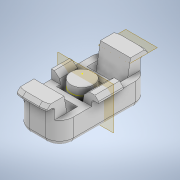
# Autodesk Inventor part: ps3buttonr1
Saved by Autodesk Inventor 2021 (Build 250183000, 183)
## iProperties
Created: 2023-05-05
Part Number: ps3buttonr1
Material: Generic
Document SubType Name: Modeling
Designer: assman
Density: 1 g/cm^3
Appearance: Default
Author: assman
## iProperties of the stored document _3DPrint.ipt
Created: 2023-05-05
Part Number: _3DPrint
Material: Generic
Document SubType Name: Modeling
Designer: assman
Density: 1 g/cm^3
Appearance: Default
Author: assman
Autodesk Inventor part; units mm, degrees
ref_plane "YZ Plane" through (0, 0, 0) normal (1, 0, 0) x (0, 1, 0)
ref_plane "XZ Plane" through (0, 0, 0) normal (0, 1, 0) x (-1, 0, 0)
sketch "Sketch1" plane through (0, 0, 0) normal (0, 1, 0) x (-1, 0, 0)
  line L0 (1.825, 9.85) -> (-1.825, 9.85)
  line L1 (-4.825, 6.85) -> (-4.825, -6.85)
  line L2 (-1.825, -9.85) -> (1.825, -9.85)
  line L3 (4.825, -6.85) -> (4.825, 6.85)
  line L4 (4.825, 9.85) -> (-4.825, -9.85) construction
  line L5 (-4.825, 9.85) -> (4.825, -9.85) construction
  arc A0 (4.825, 6.85) -> (1.825, 9.85) centre (1.825, 6.85) ccw
  arc A1 (1.825, -9.85) -> (4.825, -6.85) centre (1.825, -6.85) ccw
  arc A2 (-4.825, -6.85) -> (-1.825, -9.85) centre (-1.825, -6.85) ccw
  arc A3 (-1.825, 9.85) -> (-4.825, 6.85) centre (-1.825, 6.85) ccw
  point P0 (0, 0)
  dimension "d0" = 9.65
  dimension "d1" = 19.7
  dimension "d2" = 3
  constraints: 12 end point, 8 point on circle, 8 point on line, 8 tangent, 4 centre point, 3 equal radius, 2 midpoint, 2 parallel, 1 horizontal, 1 perpendicular
  measures "d0" distance of L5.end L4.end
  measures "d1" distance of L4.end L5.start
  measures "d2" radius of A0
extrude "Extrusion1" add sketch "Sketch1" along normal blind 5
sketch "Sketch2" plane through (0, 5, 0) normal (0, 1, 0) x (1, 0, 0)
  arc A0 (1.825, -9.85) -> (4.825, -6.85) centre (1.825, -6.85) ccw projected
  line L0 (4.825, -6.85) -> (4.825, 6.85) projected
  arc A1 (4.825, 6.85) -> (1.825, 9.85) centre (1.825, 6.85) ccw projected
  line L1 (1.825, 9.85) -> (-1.825, 9.85) projected
  arc A2 (-1.825, 9.85) -> (-4.825, 6.85) centre (-1.825, 6.85) ccw projected
  line L2 (-4.825, 6.85) -> (-4.825, -6.85) projected
  arc A3 (-4.825, -6.85) -> (-1.825, -9.85) centre (-1.825, -6.85) ccw projected
  line L3 (-1.825, -9.85) -> (1.825, -9.85) projected
  line L4 (-3.825, -8.85) -> (-3.825, 8.85)
  line L5 (-3.825, 8.85) -> (3.825, 8.85)
  line L6 (3.825, 8.85) -> (3.825, -8.85)
  line L7 (3.825, -8.85) -> (-3.825, -8.85)
  line L8 (0, -8.85) -> (0, -3.85) construction
  line L9 (0, -3.85) -> (0, -2.85) construction
  line L10 (-3.825, -2.85) -> (3.825, -2.85)
  line L11 (3.825, -2.85) -> (3.825, 2.85)
  line L12 (3.825, 2.85) -> (-3.825, 2.85)
  line L13 (-3.825, 2.85) -> (-3.825, -2.85)
  line L14 (-3.825, -2.85) -> (3.825, 2.85) construction
  line L15 (3.825, -2.85) -> (-3.825, 2.85) construction
  line L16 (-3.825, 3.85) -> (3.825, 3.85)
  line L17 (3.825, 3.85) -> (3.825, 8.85)
  line L18 (3.825, 8.85) -> (-3.825, 8.85)
  line L19 (-3.825, 8.85) -> (-3.825, 3.85)
  line L20 (-3.825, 3.85) -> (3.825, 8.85) construction
  line L21 (3.825, 3.85) -> (-3.825, 8.85) construction
  line L22 (-3.825, -8.85) -> (3.825, -8.85)
  line L23 (3.825, -8.85) -> (3.825, -3.85)
  line L24 (3.825, -3.85) -> (-3.825, -3.85)
  line L25 (-3.825, -3.85) -> (-3.825, -8.85)
  line L26 (-3.825, -8.85) -> (3.825, -3.85) construction
  line L27 (3.825, -8.85) -> (-3.825, -3.85) construction
  point P0 (0, 0)
  point P1 (0, 6.35)
  point P2 (0, -6.35)
  dimension "d5" = 1
  dimension "d6" = 5
  dimension "d8" = 1
  constraints: 48 end point, 8 midpoint, 6 parallel, 3 horizontal, 3 perpendicular, 2 point on line, 2 vertical, 3 other
  measures "d5" distance between parallel lines of L2 L4
  measures "d6" distance of L8.start L8.end
  measures "d8" distance of L8.end L9.end
extrude "Extrusion2" cut sketch "Sketch2" against normal blind 3.94 contours L4 L24 L6 L7 | L4 L12 L6 L10 | L4 L5 L6 L16
sketch "Sketch4" plane through (0, 1.06, 0) normal (0, 1, 0) x (1, 0, 0)
  line L0 (-3.825, -2.85) -> (-3.825, 2.85) construction
  line L1 (3.825, -2.85) -> (-3.825, -2.85) construction
  line L2 (3.825, 2.85) -> (3.825, -2.85) construction
  line L3 (-3.825, 2.85) -> (3.825, 2.85) construction
  circle A0 centre (0, 0) radius 2.5
  dimension "d14" = 5
  constraints: 1 centre point, 1 coincident
  measures "d14" diameter of A0
extrude "Extrusion3" add sketch "Sketch4" along normal up to surface (3.94 mm away)
sketch "Sketch5" plane through (0, 5, 0) normal (0, 1, 0) x (1, 0, 0)
  circle A0 centre (0, 0) radius 2.5 projected
thicken "Thicken1" operation add thickness 1.6 both sides no extend neighbours yes toward (0, 1, 0) faces at (1.2612, 5, 0.6619)
fillet "Fillet1" radius 1 1 edges at (-2.5, 1.06, 0)
thicken "Thicken2" operation add thickness 0.5 both sides no extend neighbours yes toward (0, 0, -1) faces at (-1.275, 3.6867, 8.85) (-3.825, 3.6867, 5.5167) (1.275, 3.6867, 3.85) (3.825, 2.3733, 5.5167)
thicken "Thicken3" operation add thickness 0.5 both sides no extend neighbours yes toward (1, 0, 0) faces at (-3.825, 2.3733, -5.5167) (1.275, 3.6867, -8.85) (3.825, 2.3733, -7.1833) (-1.275, 3.6867, -3.85)
sketch "Sketch6" plane through (1.825, 0, -9.85) normal (0, 0, -1) x (-1, 0, 0)
  line L0 (0, 0) -> (3.65, 0) construction
  line L1 (3.65, 0) -> (3.65, 5) construction
  line L2 (0, 5) -> (3.65, 5) construction
  line L3 (0, 0) -> (0, 5) construction
  line L4 (3.65, 5) -> (0, 5) construction
  line L5 (1.825, 5) -> (1.825, 0) construction
  line L6 (-0.175, 6.75) -> (3.825, 6.75) construction
  line L7 (3.825, 6.75) -> (3.825, 3.25) construction
  line L8 (3.825, 3.25) -> (-0.175, 3.25) construction
  line L9 (-0.175, 3.25) -> (-0.175, 6.75) construction
  line L10 (-0.175, 6.75) -> (3.825, 3.25) construction
  line L11 (3.825, 6.75) -> (-0.175, 3.25) construction
  line L12 (-0.175, 5) -> (5.825, 5)
  line L13 (5.825, 5) -> (5.825, 8.5)
  line L14 (5.825, 8.5) -> (-0.175, 8.5)
  line L15 (-0.175, 8.5) -> (-0.175, 5)
  dimension "d21" = 4
  dimension "d22" = 3.5
  dimension "d26" = 3.5
  constraints: 22 end point, 4 midpoint, 4 parallel, 2 horizontal, 2 perpendicular, 1 vertical
  measures "d21" distance of L7.end L8.end
  measures "d22" distance of L6.end L7.end
  measures "d26" distance of L13.end L12.end
extrude "Extrusion5" [suppressed]
sketch "Sketch8" plane through (1.825, 0, -9.85) normal (0, 0, -1) x (-1, 0, 0)
  line L0 (0, 0) -> (3.65, 0) construction
  line L1 (3.65, 0) -> (3.65, 5) construction
  line L2 (0, 0) -> (0, 5) construction
  line L3 (-0.175, 8.5) -> (-0.175, 5) projected
  line L4 (5.825, 8.5) -> (5.825, 5) projected
  line L5 (-0.175, 8.5) -> (5.825, 8.5)
  line L6 (5.825, 8.5) -> (5.825, 7.11)
  line L7 (5.825, 7.11) -> (-0.175, 7.11)
  line L8 (-0.175, 7.11) -> (-0.175, 8.5)
  line L9 (0, 5) -> (3.65, 5) projected
  point P0 (1.825, 0)
  point P1 (1.825, 5)
  point P2 (-0.175, 7.11)
  dimension "d29" = 1.39
  constraints: 8 end point, 2 parallel, 1 horizontal, 1 perpendicular, 1 point on line, 1 other
  measures "d29" distance of L5.end L6.end
extrude "Extrusion6" [suppressed]
chamfer "Chamfer1" [suppressed]
sketch "Sketch9" plane through (1.825, 0, -9.85) normal (0, 0, -1) x (-1, 0, 0)
  line L0 (0, 0) -> (0, 5) construction
  line L1 (0, 0) -> (3.65, 0) construction
  line L2 (3.65, 0) -> (3.65, 5) construction
  line L3 (1.825, 5) -> (0.825, 5)
  line L4 (0.825, 5) -> (0.825, 3)
  line L5 (0.825, 3) -> (1.825, 3)
  line L6 (1.825, 3) -> (1.825, 5)
  line L7 (5.825, 5) -> (6.825, 5)
  line L8 (6.825, 5) -> (6.825, 3)
  line L9 (6.825, 3) -> (5.825, 3)
  line L10 (5.825, 3) -> (5.825, 5)
  line L11 (0, 5) -> (3.65, 5) projected
  point P0 (1.825, 0)
  dimension "d35" = 1
  dimension "d36" = 2
  dimension "d37" = 1
  dimension "d38" = 2
  constraints: 16 end point, 4 parallel, 2 horizontal, 2 perpendicular
  measures "d35" distance of L5.end L4.end
  measures "d36" distance of L4.end L3.end
  measures "d37" distance of L8.end L9.end
  measures "d38" distance of L7.end L8.end
extrude "Extrusion7" [suppressed]
mirror "Mirror1" [suppressed]
sketch "Sketch10" plane through (4.825, 0, 6.85) normal (1, 0, 0) x (0, 0, -1)
  line L0 (0, 0) -> (13.7, 0) construction
  line L1 (13.7, 0) -> (13.7, 5) construction
  line L2 (0, 5) -> (13.7, 5) construction
  line L3 (0, 0) -> (0, 5) construction
  line L4 (8.85, 4.7327) -> (8.85, 0.7758) construction
  line L5 (6.625, 4.6249) -> (11.075, 4.6249) construction
  line L6 (11.075, 4.6249) -> (11.075, 2.1249) construction
  line L7 (11.075, 2.1249) -> (6.625, 2.1249) construction
  line L8 (6.625, 2.1249) -> (6.625, 4.6249) construction
  line L9 (6.625, 4.6249) -> (11.075, 2.1249) construction
  line L10 (11.075, 4.6249) -> (6.625, 2.1249) construction
  line L11 (6.625, 5) -> (11.075, 5)
  line L12 (11.075, 5) -> (11.075, 7.5)
  line L13 (11.075, 7.5) -> (6.625, 7.5)
  line L14 (6.625, 7.5) -> (6.625, 5)
  point P0 (6.85, 0)
  point P1 (8.85, 3.3749)
  dimension "d41" = 4.45
  dimension "d42" = 2.5
  dimension "d43" = 4.45
  dimension "d44" = 2.5
  constraints: 22 end point, 4 parallel, 3 point on line, 2 horizontal, 2 midpoint, 2 perpendicular, 1 vertical
  measures "d41" distance of L6.end L7.end
  measures "d42" distance of L5.end L6.end
  measures "d43" distance of L13.end L12.end
  measures "d44" distance of L12.end L11.end
extrude "Extrusion8" [suppressed]
sketch "Sketch11" plane through (4.825, 0, 6.85) normal (1, 0, 0) x (0, 0, -1)
  line L0 (0, 0) -> (13.7, 0) construction
  line L1 (13.7, 0) -> (13.7, 5) construction
  line L2 (0, 5) -> (13.7, 5) construction
  line L3 (0, 0) -> (0, 5) construction
  line L4 (6.625, 5) -> (5.825, 5)
  line L5 (5.825, 5) -> (5.825, 3)
  line L6 (5.825, 3) -> (6.625, 3)
  line L7 (6.625, 3) -> (6.625, 5)
  line L8 (11.075, 5) -> (11.875, 5)
  line L9 (11.875, 5) -> (11.875, 3)
  line L10 (11.875, 3) -> (11.075, 3)
  line L11 (11.075, 3) -> (11.075, 5)
  point P0 (6.85, 0)
  dimension "d47" = 0.8
  dimension "d48" = 2
  dimension "d49" = 0.8
  dimension "d50" = 2
  constraints: 16 end point, 4 parallel, 2 horizontal, 2 perpendicular
  measures "d47" distance of L6.end L5.end
  measures "d48" distance of L5.end L4.end
  measures "d49" distance of L9.end L10.end
  measures "d50" distance of L8.end L9.end
extrude "Extrusion9" [suppressed]
sketch "Sketch12" plane through (4.825, 0, 6.85) normal (1, 0, 0) x (0, 0, -1)
  line L0 (0, 5) -> (13.7, 5) construction
  line L1 (0, 0) -> (0, 5) construction
  line L2 (0, 0) -> (13.7, 0) construction
  line L3 (13.7, 0) -> (13.7, 5) construction
  line L4 (6.625, 7.5) -> (11.075, 7.5) projected
  line L5 (11.075, 3) -> (11.075, 7.5) projected
  line L6 (6.625, 7.5) -> (11.075, 7.5)
  line L7 (11.075, 7.5) -> (11.075, 6)
  line L8 (11.075, 6) -> (6.625, 6)
  line L9 (6.625, 6) -> (6.625, 7.5)
  point P0 (6.85, 0)
  dimension "d53" = 1.5
  constraints: 8 end point, 2 parallel, 1 horizontal, 1 perpendicular, 1 point on line
  measures "d53" distance of L6.end L7.end
extrude "Extrusion10" [suppressed]
chamfer "Chamfer2" [suppressed]
sketch "Sketch13" plane through (-4.825, 0, -6.85) normal (-1, 0, 0) x (0, 0, 1)
  line L0 (0, 0) -> (13.7, 0) construction
  line L1 (13.7, 0) -> (13.7, 5) construction
  line L2 (0, 5) -> (13.7, 5) construction
  line L3 (0, 0) -> (0, 5) construction
  line L4 (0, 5) -> (13.7, 5) construction
  line L5 (6.85, 5) -> (6.85, 0) construction
  line L6 (5.35, 4.8143) -> (8.35, 4.8143) construction
  line L7 (8.35, 4.8143) -> (8.35, 2.8143) construction
  line L8 (8.35, 2.8143) -> (5.35, 2.8143) construction
  line L9 (5.35, 2.8143) -> (5.35, 4.8143) construction
  line L10 (5.35, 4.8143) -> (8.35, 2.8143) construction
  line L11 (8.35, 4.8143) -> (5.35, 2.8143) construction
  line L12 (5.35, 5) -> (10.35, 5)
  line L13 (10.35, 5) -> (10.35, 7)
  line L14 (10.35, 7) -> (5.35, 7)
  line L15 (5.35, 7) -> (5.35, 5)
  point P0 (6.85, 3.8143)
  dimension "d59" = 3
  dimension "d60" = 2
  dimension "d61" = 2
  constraints: 22 end point, 4 parallel, 3 midpoint, 3 point on line, 2 horizontal, 2 perpendicular, 1 vertical
  measures "d59" distance of L7.end L8.end
  measures "d60" distance of L6.end L7.end
  measures "d61" distance of L13.end L12.end
extrude "Extrusion11" [suppressed]
sketch "Sketch15" plane through (4.825, 0, 6.85) normal (1, 0, 0) x (0, 0, -1)
  line L0 (0, 0) -> (13.7, 0) construction
  line L1 (13.7, 0) -> (13.7, 5) construction
  line L2 (0, 5) -> (13.7, 5) construction
  line L3 (0, 0) -> (0, 5) construction
  line L4 (4.35, 6.6) -> (9.35, 6.6) construction
  line L5 (4.35, 2.06) -> (9.35, 2.06) construction
  line L6 (4, 5) -> (4, 1.06) construction
  line L7 (9.7, 5) -> (4, 5) construction
  line L8 (9.7, 5) -> (9.7, 1.06) construction
  line L9 (4.625, 6) -> (9.075, 6) construction
  line L10 (9.075, 6) -> (9.075, 4) construction
  line L11 (9.075, 4) -> (4.625, 4) construction
  line L12 (4.625, 4) -> (4.625, 6) construction
  line L13 (9.7, 5) -> (4, 5) construction
  line L14 (4.625, 6) -> (9.075, 4) construction
  line L15 (9.075, 6) -> (4.625, 4) construction
  line L16 (4.625, 5) -> (9.075, 5)
  line L17 (9.075, 5) -> (9.075, 7.5)
  line L18 (9.075, 7.5) -> (4.625, 7.5)
  line L19 (4.625, 7.5) -> (4.625, 5)
  line L20 (9.7, 1.06) -> (4, 1.06) projected
  point P0 (6.85, 0)
  point P1 (6.85, 5)
  dimension "d70" = 4.45
  dimension "d71" = 2
  dimension "d72" = 2.5
  dimension "d97" = 4.45
  constraints: 20 end point, 4 midpoint, 4 parallel, 2 horizontal, 2 perpendicular, 1 point on line
  measures "d70" distance of L10.end L11.end
  measures "d71" distance of L9.end L10.end
  measures "d72" distance of L17.end L16.end
  measures "d97" distance of L17.end L18.end
extrude "Extrusion13" add sketch "Sketch15" against normal up to surface (1 mm away)
thicken "Thicken4" operation add thickness 0.5 both sides no extend neighbours yes toward (-1, 0, 0) faces at (3.825, 2.3733, -0.7417)
draft "FaceDraft1" angle 10 pull direction (0, 1, 0) faces at (3.325, 3.6918, 0) fixed edges at (3.325, 7.5, 0)
sketch "Sketch16" plane through (-4.825, 0, -6.85) normal (-1, 0, 0) x (0, 0, 1)
  line L0 (0, 0) -> (13.7, 0) construction
  line L1 (13.7, 0) -> (13.7, 5) construction
  line L2 (0, 5) -> (13.7, 5) construction
  line L3 (0, 0) -> (0, 5) construction
  line L4 (9.7, 5) -> (4, 5) construction
  line L5 (9.7, 5) -> (9.7, 1.06) construction
  line L6 (9.7, 1.06) -> (4, 1.06) construction
  line L7 (4, 5) -> (4, 1.06) construction
  line L8 (5.35, 6) -> (8.35, 6) construction
  line L9 (8.35, 6) -> (8.35, 4) construction
  line L10 (8.35, 4) -> (5.35, 4) construction
  line L11 (5.35, 4) -> (5.35, 6) construction
  line L12 (9.7, 5) -> (4, 5) construction
  line L13 (5.35, 6) -> (8.35, 4) construction
  line L14 (8.35, 6) -> (5.35, 4) construction
  line L15 (5.35, 5) -> (8.35, 5)
  line L16 (8.35, 5) -> (8.35, 7)
  line L17 (8.35, 7) -> (5.35, 7)
  line L18 (5.35, 7) -> (5.35, 5)
  point P0 (6.85, 0)
  point P1 (6.85, 5)
  dimension "d78" = 3
  dimension "d79" = 2
  dimension "d80" = 2
  constraints: 20 end point, 4 midpoint, 4 parallel, 2 horizontal, 2 perpendicular, 1 point on line
  measures "d78" distance of L9.end L10.end
  measures "d79" distance of L8.end L9.end
  measures "d80" distance of L16.end L15.end
extrude "Extrusion14" add sketch "Sketch16" against normal up to surface (1 mm away)
thicken "Thicken5" operation add thickness 0.5 both sides no extend neighbours yes toward (1, 0, 0) faces at (-3.825, 2.3733, 0.5)
thicken "Thicken6" operation add thickness 0.5 both sides no extend neighbours yes toward (1, 0, 0) faces at (-3.325, 3.6867, 0.3643)
draft "FaceDraft2" angle 10 pull direction (0, 1, 0) faces at (-2.825, 3.7741, 0) fixed edges at (-2.825, 5, -2.175)
sketch "Sketch18" plane through (0, 5, 0) normal (0, 1, 0) x (1, 0, 0)
  line L0 (-3.325, 8.35) -> (3.325, 8.35) projected
  arc A0 (4.825, 6.85) -> (1.825, 9.85) centre (1.825, 6.85) ccw projected
  line L1 (1.825, 9.85) -> (-1.825, 9.85) projected
  arc A1 (-1.825, 9.85) -> (-4.825, 6.85) centre (-1.825, 6.85) ccw projected
  line L2 (-3.325, 8.35) -> (3.325, 8.35) projected
  line L3 (3.325, 8.35) -> (3.325, 9.4481)
  arc A2 (4.825, 6.85) -> (1.825, 9.85) centre (1.825, 6.85) ccw projected
  line L4 (-3.325, 8.35) -> (-3.325, 9.4481)
  point P0 (0, 0)
  constraints: 4 end point, 2 point on circle, 1 parallel, 1 vertical
extrude "Extrusion15" add sketch "Sketch18" along normal blind 3.5
thicken "Thicken7" operation add thickness 1 both sides no extend neighbours yes toward (0, 0, 1) faces at (-1.1083, 2.3733, -8.35)
draft "FaceDraft3" angle 10 pull direction (0, 1, 0) faces at (-1.1083, 2.3733, -7.35) fixed edges at (0, 8.5, -7.35)
ref_plane "Work Plane1" through (0, 7.5, 0) normal (0, 1, 0) x (1, 0, 0)
sketch "Sketch19" plane through (0, 7.5, 0) normal (0, 1, 0) x (1, 0, 0)
  point P0 (0, 0)
split body "Split1" result two bodies by plane through (0, 7.5, 0) normal (0, 1, 0) first body at (-0.6083, 8, -8.0658)
thicken "Thicken8" operation add thickness 1.5 both sides no extend neighbours yes toward (0.3960798, 0, -0.9182161) bodies 2 faces at (3.0132, 7.8333, -9.6046) (-0.6083, 8.1667, -9.85) (-1.9994, 7.8333, -9.8449)
combine bodies "Combine1" operation type add bodies to combine 2 3
fillet "Fillet3" radius 0.5 1 edges at (2.6015, 7.5, -9.7478)
thicken "Thicken9" operation add thickness 0.5 both sides no extend neighbours yes toward (0, 0, 1) bodies 2 faces at (3.6781, 5.8333, 2.225)
thicken "Thicken10" operation add thickness 0.5 both sides no extend neighbours yes toward (0, 0, -1) bodies 2 faces at (3.6781, 5.8333, -2.225)
thicken "Thicken11" operation add thickness 0.5 both sides no extend neighbours yes toward (0, 0, 1) bodies 2 faces at (-3.6092, 5.6667, 1.5)
thicken "Thicken12" operation add thickness 0.5 both sides no extend neighbours yes toward (0, 0, -1) bodies 2 faces at (-3.6583, 5.6667, -1.5)
sketch "Sketch20" plane through (4.825, 0, 6.85) normal (1, 0, 0) x (0, 0, -1)
  line L0 (0, 0) -> (13.7, 0) construction
  line L1 (13.7, 0) -> (13.7, 5) construction
  line L2 (9.575, 5) -> (13.7, 5) construction
  line L3 (9.575, 5) -> (9.575, 7.5) construction
  line L4 (9.575, 7.5) -> (4.125, 7.5) construction
  line L5 (4.125, 7.5) -> (4.125, 5) construction
  line L6 (0, 5) -> (4.125, 5) construction
  line L7 (0, 0) -> (0, 5) construction
  line L8 (4.125, 7.5) -> (9.575, 7.5) projected
  line L9 (4.125, 7.5) -> (9.575, 7.5)
  line L10 (9.575, 7.5) -> (9.575, 6.3)
  line L11 (9.575, 6.3) -> (4.125, 6.3)
  line L12 (4.125, 6.3) -> (4.125, 7.5)
  point P0 (6.85, 0)
  dimension "d106" = 1.2
  constraints: 8 end point, 2 parallel, 1 horizontal, 1 perpendicular, 1 point on line
  measures "d106" distance of L9.end L10.end
extrude "Extrusion16" add sketch "Sketch20" along normal blind 1.5 bodies 2
fillet "Fillet4" radius 0.572 1 edges at (4.825, 6.3, 0)
chamfer "Chamfer3" distance 0.8 angle 45 1 edges at (6.325, 7.5, 0)
chamfer "Chamfer4" distance 0.7 angle 45 3 edges at (0, 8.5, -11.35) (-2.586, 8.5, -11.2852) (2.586, 8.5, -11.2852)
ref_plane "Work Plane2" through (0, 0, 0) normal (0, 0, 1) x (1, 0, 0)
split "Split2" plane through (0, 0, 0) removes the side toward (0, 0, 1) bodies 2
mirror "Mirror2" about plane through (0, 0, 0) normal (0, 0, 1) bodies 2
sketch "Sketch14" plane through (0, 0, 0) normal (0, -1, 0) x (1, 0, 0)
  line L0 (-3.0082, -2.7578) -> (-3.0082, 2.7578) construction
  line L1 (-3.0082, 2.7578) -> (3.0082, 2.7578) construction
  line L2 (3.0082, 2.7578) -> (3.0082, -2.7578) construction
  line L3 (3.0082, -2.7578) -> (-3.0082, -2.7578) construction
  line L4 (-1.5514, -1.4223) -> (1.5514, 1.4223) construction
  line L5 (1.5514, -1.4223) -> (-1.5514, 1.4223) construction
  line L6 (-3.0082, 1.3063) -> (3.0082, 1.3063)
  line L7 (3.0082, 1.3063) -> (3.0082, -0.3557)
  line L8 (3.0082, -0.3557) -> (-0.9363, -0.3557)
  spline S0 degree 2 poles (-0.9363, -0.3557) (-0.629, -0.7599) (-0.2533, -1.5112) (-0.0768, -2.0804) knots 0 0 0 1 2 2 2
  line L9 (-0.0768, -2.0804) -> (-1.4258, -2.0804)
  spline S1 degree 2 poles (-1.4258, -2.0804) (-1.6934, -1.2437) (-2.4504, -0.3159) (-3.0082, -0.0541) knots 0 0 0 1 2 2 2
  line L10 (-3.0082, -0.0541) -> (-3.0082, 1.3063)
  point P0 (0, 0)
  point P1 (0, 0)
  point P2 (0, 0)
  constraints: 4 end point, 2 midpoint, 1 coincident, 2 other
extrude "Extrusion12" cut sketch "Sketch14" against normal blind 0.2 bodies 2
fillet "Fillet5" radius 1 8 edges at (-3.9463, 0, -8.9713) (0, 0, -9.85) (3.9463, 0, -8.9713) (4.825, 0, 0) (3.9463, 0, 8.9713) (0, 0, 9.85) (-3.9463, 0, 8.9713) (-4.825, 0, 0)
chamfer "Chamfer5" distance 1 angle 45 2 edges at (-3.1777, 7, 0) (3.325, 7.5, 0)
body "Solid2"
